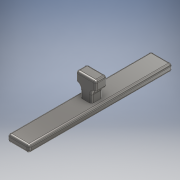
# Autodesk Inventor part: Latch Slide
Saved by Autodesk Inventor 2018 (Build 220112000, 112)
## iProperties
Created: 2018-10-16
Part Number: Latch Slide
Material: Steel
Document SubType Name: Modeling
Designer: P301319
Density: 7.85 g/cm^3
Appearance: Semi-Polished
Author: P301319
Autodesk Inventor part; units mm, degrees
ref_plane "YZ Plane" through (0, 0, 0) normal (1, 0, 0) x (0, 1, 0)
ref_plane "XZ Plane" through (0, 0, 0) normal (0, 1, 0) x (-1, 0, 0)
ref_plane "XY Plane" through (0, 0, 0) normal (0, 0, 1) x (1, 0, 0)
sketch "Sketch1" plane through (0, 0, 0) normal (0, 1, 0) x (-1, 0, 0)
  line L0 (0, 0) -> (-15, 0)
  line L1 (-15, 0) -> (-15, -5)
  line L2 (-15, -5) -> (0, -5)
  line L3 (0, -5) -> (0, 0)
  dimension "d2" = 15
  dimension "d3" = 5
  constraints: 8 end point, 2 parallel, 1 horizontal, 1 perpendicular
  measures "d2" distance between parallel lines of L1 L3
  measures "d3" distance between parallel lines of L0 L2
extrude "Extrusion1" add sketch "Sketch1" along normal blind 100
sketch "Sketch2" plane through (0, 0, 0) normal (0, 0, 1) x (1, 0, 0)
  line L0 (3.5, 55) -> (11.5, 55)
  line L1 (11.5, 55) -> (11.5, 47)
  line L2 (11.5, 47) -> (3.5, 47)
  line L3 (3.5, 47) -> (3.5, 55)
  line L4 (0, 0) -> (15, 0) projected
  point P0 (7.5, 47)
  point P1 (7.5, 0)
  dimension "d6" = 8
  dimension "d7" = 8
  dimension "d8" = 55
  constraints: 8 end point, 2 midpoint, 2 parallel, 1 horizontal, 1 perpendicular, 1 vertical alignment
  measures "d6" distance of L1.end L2.end
  measures "d7" distance of L0.end L1.end
  measures "d8" distance between parallel lines of L4 L0
extrude "Extrusion2" add sketch "Sketch2" along normal blind 15
sketch "Sketch3" plane through (11.5, 47, 0) normal (1, 0, 0) x (0, 0, -1)
  line L0 (0, 8) -> (-15, 8) projected
  line L1 (-15, 8) -> (-8, 8)
  line L2 (-8, 8) -> (-8, 0)
  line L3 (-8, 0) -> (-15, 0)
  line L4 (-15, 0) -> (-15, 8)
  point P0 (0, -47)
  dimension "d11" = 7
  dimension "d12" = 8
  constraints: 8 end point, 2 parallel, 1 horizontal, 1 perpendicular
  measures "d11" distance of L2.end L3.end
  measures "d12" distance of L1.end L2.end
extrude "Extrusion3" add sketch "Sketch3" along normal blind 3
sketch "Sketch4" plane through (3.5, 47, 0) normal (-1, 0, 0) x (0, 0, 1)
  line L0 (15, 8) -> (15, 0) projected
  line L1 (15, 8) -> (8, 8)
  line L2 (8, 8) -> (8, 0)
  line L3 (8, 0) -> (15, 0)
  line L4 (15, 0) -> (15, 8)
  point P0 (0, -47)
  dimension "d15" = 7
  dimension "d16" = 8
  constraints: 8 end point, 2 parallel, 1 horizontal, 1 perpendicular
  measures "d15" distance of L3.end L2.end
  measures "d16" distance of L2.end L1.end
extrude "Extrusion4" add sketch "Sketch4" along normal blind 3
fillet "Fillet1" radius 3 2 edges at (3.5, 51, 8) (11.5, 51, 8)
fillet "Fillet2" radius 1.5 24 edges at (14.5, 47, 8) (14.5, 51, 8) (14.5, 55, 8) (14.4999, 51, 8) (11.5, 55, 2.5) (12.3787, 55, 7.1213) (14.5, 55, 11.5) (12.3787, 47, 7.1213) (11.5, 47, 2.5) (3.5, 47, 2.5) (0.5001, 47, 8) (2.6213, 47, 7.1213) (0.5, 47, 11.5) (14.5, 47, 11.5) (7.5, 47, 15) (7.5, 55, 15) (0.5, 51, 15) (14.5, 51, 15) (0.5001, 55, 8) (0.5001, 51, 8) (0.5, 51, 8) (3.5, 55, 2.5) (2.6213, 55, 7.1213) (0.5, 55, 11.5)
fillet "Fillet3" radius 1.5 12 edges at (15, 50, 0) (0, 50, 0) (0, 50, -5) (15, 50, -5) (7.5, 100, 0) (15, 100, -2.5) (7.5, 100, -5) (0, 100, -2.5) (7.5, 0, -5) (0, 0, -2.5) (7.5, 0, 0) (15, 0, -2.5)
body "Solid1"
